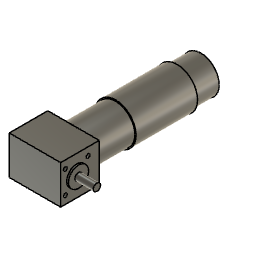
BG42-4266 (Autodesk Fusion 360 design; units mm, degrees)
Autodesk Fusion 360 part; units mm, degrees
sketch "스케치1" plane through (0, 0, 0) normal (0, 1, 0) x (1, 0, 0)
  line L0 (28, -21) -> (-28, -21)
  line L1 (-28, -21) -> (-28, 21)
  line L2 (-28, 21) -> (28, 21)
  line L3 (28, 21) -> (28, -21)
  line L4 (28, -21) -> (-28, 21) construction
  line L5 (-28, -21) -> (28, 21) construction
  dimension "d1" = 56
  dimension "d2" = 42
  constraint horizontal L0
  constraint perpendicular L0 L1
  constraint parallel L0 L2
  constraint parallel L1 L3
  constraint coincident L4 origin
  constraint coincident L5 origin
  measures "d1" distance of L1.end L2.end
  measures "d2" distance of L0.end L1.end
extrude "돌출1" add sketch "스케치1" along normal blind 42
sketch "스케치2" plane through (0, 42, 0) normal (0, 1, 0) x (-1, 0, 0)
  line L0 (-28, -21) -> (28, -21)
  line L1 (28, -21) -> (28, 21)
  line L2 (28, 21) -> (-28, 21)
  line L3 (-28, 21) -> (-28, -21)
  circle A0 centre (0, 0) radius 21
  dimension "d5" = 42
  constraint coincident A0.centre origin
  measures "d5" diameter of A0
extrude "돌출2" add sketch "스케치2" along normal blind 45.9 contours A0
sketch "스케치3" plane through (0, 87.9, 0) normal (0, 1, 0) x (-1, 0, 0)
  circle A0 centre (0, 0) radius 21
  circle A1 centre (0, 0) radius 22.3
  dimension "d8" = 44.6
  constraint coincident A0.centre A1.centre
  measures "d8" diameter of A1
extrude "돌출3" add sketch "스케치3" along normal blind 67 contours A0 | A1
sketch "스케치4" plane through (0, 154.9, 0) normal (0, 1, 0) x (-1, 0, 0)
  circle A0 centre (0, 0) radius 22.3
  circle A1 centre (0, 0) radius 20
  dimension "d11" = 40
  constraint coincident A0.centre A1.centre
  measures "d11" diameter of A1
extrude "돌출4" add sketch "스케치4" along normal blind 25.9 contours A1
sketch "스케치5" plane through (28, 0, 0) normal (1, 0, 0) x (0, 1, 0)
  line L0 (0, 21) -> (0, -21)
  line L1 (0, -21) -> (42, -21)
  line L2 (42, -21) -> (42, 21)
  line L3 (42, 21) -> (0, 21)
  line L4 (0, 0) -> (17.5, 0)
  circle A0 centre (17.5, 0) radius 17.5
  line L5 (17.5, 0) -> (5.1256, 12.3744)
  line L6 (17.5, 0) -> (35, 0) construction
  circle A1 centre (5.1256, 12.3744) radius 2.1
  circle A2 centre (5.1256, -12.3744) radius 2.1
  circle A3 centre (29.8744, -12.3744) radius 2.1
  circle A4 centre (29.8744, 12.3744) radius 2.1
  circle A5 centre (17.5, 0) radius 11
  circle A6 centre (17.5, 0) radius 4
  line L7 (17.5, 0) -> (17.5, -21)
  dimension "d14" = 17.5
  dimension "d15" = 135
  dimension "d16" = 4.2
  dimension "d18" = 360
  dimension "d19" = 22
  dimension "d20" = 8
  dimension "d27" = 21
  constraint coincident L4.start origin
  constraint perpendicular L0 L4
  constraint coincident L4.end A0.centre
  constraint coincident L4.start A0
  constraint horizontal L6
  constraint coincident A0 L5.end
  constraint coincident L5.end A1.centre
  constraint concentric A0 A5
  constraint concentric A0 A6
  constraint coincident L1 L7.end
  constraint perpendicular L1 L7
  measures "d14" distance of L4.start L4.end
  measures "d15" angle of L5 L6
  measures "d16" diameter of A1
  measures "d19" diameter of A5
  measures "d20" diameter of A6
  measures "d27" distance of L4.end L7.end
extrude "돌출5" add sketch "스케치5" along normal blind 2 contours L4 L5 A5 A6 | L4 A5 A6 L7 | L5 A5 A6 L7
extrude "돌출6" add sketch "스케치5" along normal blind 22 contours L4 L5 A6 | L4 A6 L7 | L5 A6 L7
extrude "돌출7" cut sketch "스케치5" against normal blind 7 contours A0 A1 | A0 L5 A1 | A0 A2 | A0 A2 | A0 L5 A1 | A0 A4 | A0 A4 | A0 A3 | A0 A3
